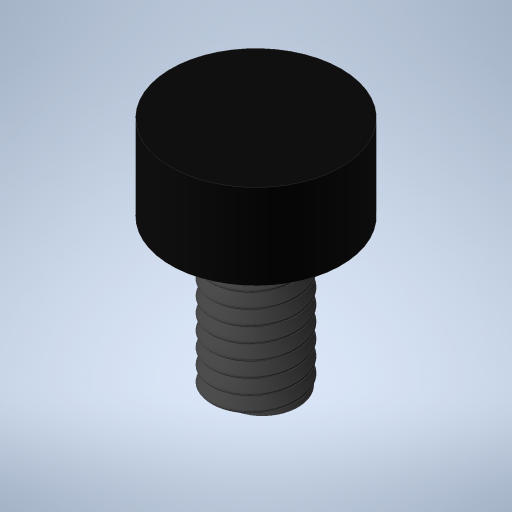
# Autodesk Inventor part: restrainer_back_screw
Saved by Autodesk Inventor 2023 (Build 270158000, 158)
## iProperties
Created: 2022-11-01
Part Number: restrainer_back_screw
Material: Generic
Document SubType Name: Modeling
Designer: Admin
Density: 1 g/cm^3
Appearance: Default
Author: Admin
Autodesk Inventor part; units mm, degrees
ref_plane "YZ Plane" through (0, 0, 0) normal (1, 0, 0) x (0, 1, 0)
ref_plane "XZ Plane" through (0, 0, 0) normal (0, 1, 0) x (-1, 0, 0)
ref_plane "XY Plane" through (0, 0, 0) normal (0, 0, 1) x (1, 0, 0)
sketch "Sketch1" plane through (0, 0, 0) normal (1, 0, 0) x (0, 1, 0)
  line L0 (0, 0) -> (-7, 0)
  line L1 (-7, 0) -> (-7, -2)
  line L2 (-7, -2) -> (0, -2)
  line L3 (0, -2) -> (0, 0)
  line L4 (0, 0) -> (4, 0)
  line L5 (4, 0) -> (4, -4)
  line L6 (4, -4) -> (0, -4)
  line L7 (0, -4) -> (0, 0)
  point P0 (0, -2)
  dimension "d0" = 7
  dimension "d1" = 2
  dimension "d2" = 4
  dimension "d3" = 4
  constraints: 16 end point, 4 parallel, 2 horizontal, 2 perpendicular
  measures "d0" distance of L2.end L1.end
  measures "d1" distance of L0.end L1.end
  measures "d2" distance of L5.end L6.end
  measures "d3" distance of L4.end L5.end
revolve "Revolution1" add sketch "Sketch1" angle 360 about axis through (0, 0, 0) along (0, 1, 0)
thread "Thread3" size "M4x0.7" class "6g" standard "ANSI Metric M Profile" length 7
sketch "Sketch9" plane through (0, -7, 0) normal (-1, 0, 0) x (0, 0, 1)
  line L0 (2, 0) -> (2, 7)
  line L1 (2, 7) -> (1.481, 7)
  line L2 (1.481, 7) -> (1.481, 0)
  line L3 (1.481, 0) -> (2, 0)
  line L4 (0, -3.1161) -> (0, 13.3527) projected
  constraints: 8 end point
revolve "Revolution6" cut sketch "Sketch9" angle 360 about axis through (0, -7, 0) along (0, 1, 0)
sketch "Sketch10" plane through (0, -7, 0) normal (-1, 0, 0) x (0, 0, 1)
  line L0 (2, 0) -> (2, 7)
  line L1 (2, 7) -> (1.481, 7)
  line L2 (1.481, 7) -> (1.481, 0)
  line L3 (1.481, 0) -> (2, 0)
  line L4 (0, -3.1161) -> (0, 13.3527) projected
  constraints: 8 end point
revolve "Revolution7" add sketch "Sketch10" angle 360 about axis through (0, -7, 0) along (0, 1, 0) separate body
sketch "Sketch8" plane through (0, -7, 0) normal (1, 0, 0) x (0, 1, 0)
  line L0 (-0.4084, -1.5165) -> (-0.3501, -1.5165) construction
  line L1 (0.0582, -1.9648) -> (-0.0001, -2.0768) construction
  line L2 (-0.7001, -2.0768) -> (-0.7584, -1.9648) construction
  line L3 (-0.2918, -1.5165) -> (-0.3501, -1.4045) construction
  line L4 (-0.3501, -1.4045) -> (-0.4084, -1.5165) construction
  line L5 (-0.7001, -2.0768) -> (-0.6418, -1.9648) construction
  line L6 (-0.2918, -1.5165) -> (-0.0584, -1.9648)
  line L7 (-0.7584, -1.9648) -> (-0.6418, -1.9648) construction
  arc A0 (-0.7584, -1.9648) -> (-0.7001, -2.0002) centre (-0.7001, -1.9344) ccw construction
  line L8 (0.0582, -1.9648) -> (-0.0584, -1.9648) construction
  line L9 (-0.7001, -2.0768) -> (-0.7001, -1.9648) construction
  line L10 (-0.0001, -2.0768) -> (-0.0001, -1.9648) construction
  line L11 (-0.3501, -1.4045) -> (-0.3501, -1.4811) construction
  line L12 (-0.7001, -2.0002) -> (-0.0001, -2.0002)
  arc A1 (-0.7001, -2.0002) -> (-0.6418, -1.9648) centre (-0.7001, -1.9344) ccw
  line L13 (-0.0584, -1.9648) -> (-0.0001, -2.0768) construction
  line L14 (-0.6418, -1.9648) -> (-0.4084, -1.5165)
  line L15 (-0.0001, -0.0002) -> (-0.0001, 0.0177)
  line L16 (-0.0001, 0.0177) -> (-0.0001, -0.0002)
  line L17 (-0.0001, -0.0002) -> (0.0334, -0.0002)
  arc A2 (-0.0584, -1.9648) -> (-0.0001, -2.0002) centre (-0.0001, -1.9344) ccw
  arc A3 (-0.0001, -2.0002) -> (0.0582, -1.9648) centre (-0.0001, -1.9344) ccw construction
  arc A4 (-0.3501, -1.4811) -> (-0.4084, -1.5165) centre (-0.3501, -1.5469) ccw
  arc A5 (-0.2918, -1.5165) -> (-0.3501, -1.4811) centre (-0.3501, -1.5469) ccw
  line L18 (-0.3501, -1.4811) -> (-0.3501, -1.5165) construction
  line L19 (-0.3501, -1.5165) -> (-0.2918, -1.5165) construction
  dimension "d49" = 55
  dimension "d50" = 0.1121
  dimension "d51" = 0.1121
  dimension "Sketch8_ThreadOffset" = 0
  dimension "Sketch8_MajorRadius" = 2
  dimension "d54" = 0.7
  dimension "Sketch8_MinorRadius" = 1.481
  constraints: 40 end point, 12 point on circle, 10 parallel, 8 tangent, 6 centre point, 6 collinear, 2 midpoint, 2 point on line, 1 horizontal, 1 perpendicular, 3 other
  measures "d49" angle of L6 L14
  measures "d50" distance of L3.end L0.end
  measures "d51" distance of L1.end L10.end
  measures "Sketch8_ThreadOffset" distance between parallel lines of L15 L10
  measures "Sketch8_MajorRadius" distance from line of L12 L15.start
  measures "d54" distance from line of L1.end L9
  measures "Sketch8_MinorRadius" distance edge to line of A5 L17
coil "Coil3" sketch "Sketch8" operation cut axis through (0, -7, 0) along (0, 1, 0) pitch 0.7007 turns 11.988012 hand right bodies 2
equation "\"d49\" = d56"
equation "\"d50\" = 0.160083 * Sketch8_Pitch"
equation "\"d51\" = 0.160083 * Sketch8_Pitch"
equation "\"d54\" = Sketch8_Pitch"
equation "\"d14\" = 55deg"
equation "\"Sketch2_Pitch\" = 0.7"
equation "\"d35\" = 55deg"
equation "\"Sketch5_Pitch\" = 0.7"
equation "\"d56\" = 55deg"
equation "\"Sketch8_Pitch\" = 0.7"
body "Solid1"
body "Solid4"
